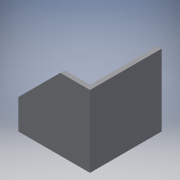
# Autodesk Inventor part: bottom left rail gusset
Saved by Autodesk Inventor 2016 (Build 200138000, 138)
## iProperties
Created: 2016-02-08
Part Number: bottom left rail gusset
Material: Aluminum 6061
Document SubType Name: Modeling
Designer: gus
Density: 2.7 g/cm^3
Appearance: Aluminum - Flat
Mass: 35.9431 g
Surface Area: 95.0795 cm^2
Volume: 13.3122 cm^3
Author: gus
Autodesk Inventor part; units mm, degrees
ref_plane "YZ Plane" through (0, 0, 0) normal (1, 0, 0) x (0, 1, 0)
ref_plane "XZ Plane" through (0, 0, 0) normal (0, 1, 0) x (-1, 0, 0)
ref_plane "XY Plane" through (0, 0, 0) normal (0, 0, 1) x (1, 0, 0)
sketch "Sketch1" plane through (0, 0, 0) normal (0, 0, 1) x (1, 0, 0)
  line L0 (0, 0) -> (0, 21.042)
  line L1 (0, 21.042) -> (29.758, 50.8)
  line L2 (29.758, 50.8) -> (50.8, 50.8)
  line L3 (50.8, 50.8) -> (50.8, 0)
  line L4 (50.8, 0) -> (0, 0)
  dimension "d0" = 50.8
  dimension "d2" = 50.8
  dimension "d3" = 50.8
  dimension "d4" = 135
  constraints: 10 end point, 3 perpendicular, 1 vertical
  measures "d0" distance of L3.end L0.start
  measures "d2" distance of L2.end L3.end
  measures "d3" distance from line of L3.end L1
  measures "d4" angle of L2 L1
extrude "Extrusion1" add sketch "Sketch1" along normal blind 3.175
sketch "Sketch2" plane through (0, 0, 3.175) normal (0, 0, 1) x (1, 0, 0)
  line L0 (50.8, 0) -> (50.8, 50.8) projected
  line L1 (0, 0) -> (50.8, 0) projected
  line L2 (50.8, 50.8) -> (47.625, 50.8)
  line L3 (47.625, 50.8) -> (47.625, 0)
  line L4 (47.625, 0) -> (50.8, 0)
  line L5 (50.8, 0) -> (50.8, 50.8)
  dimension "d7" = 3.175
  constraints: 8 end point, 2 parallel, 1 horizontal, 1 perpendicular, 1 point on line
  measures "d7" distance between parallel lines of L3 L0
extrude "Extrusion2" add sketch "Sketch2" against normal blind 50.8
sketch "Sketch3" plane through (50.8, 0, 3.175) normal (1, 0, 0) x (0, 0, -1)
  circle A0 centre (38.1, 36.9316) radius 3.3734
  circle A1 centre (12.7, 36.9316) radius 3.3734
  line L0 (0, 50.8) -> (50.8, 50.8) projected
  line L1 (0, 0) -> (0, 50.8) projected
  point P0 (3.175, 0)
  dimension "d10" = 6.7469
  dimension "d11" = 6.7469
  dimension "d12" = 13.8684
  dimension "d13" = 13.8684
  dimension "d14" = 12.7
  dimension "d15" = 25.4
  constraints: 2 centre point
  measures "d10" diameter of A0
  measures "d11" diameter of A1
  measures "d12" distance from line of A1.centre L0
  measures "d13" distance from line of L0 A0.centre
  measures "d14" distance from line of L1 A1.centre
  measures "d15" distance of A0.centre A1.centre
extrude "Extrusion3" cut sketch "Sketch3" against normal blind 3.175
sketch "Sketch4" plane through (0, 0, 0) normal (0, 0, -1) x (-1, 0, 0)
  line L0 (0, 0) -> (0, 21.042) projected
  line L1 (0, 21.042) -> (-21.042, 0)
  line L2 (-47.625, 0) -> (0, 0) projected
  line L3 (0, 21.042) -> (-29.758, 50.8) projected
  line L4 (0, 21.042) -> (0, 0)
  line L5 (-21.042, 0) -> (0, 0)
  circle A0 centre (-20.7624, 23.8439) radius 3.3734
  circle A1 centre (-38.7229, 41.8044) radius 3.3734
  dimension "d18" = 16.6624
  dimension "d19" = 12.7
  dimension "d20" = 12.7
  dimension "d21" = 6.7469
  dimension "d22" = 25.4
  constraints: 6 end point, 2 centre point, 1 equal radius, 1 horizontal, 1 perpendicular, 1 point on line, 1 vertical
  measures "d18" distance from line of A0.centre L1
  measures "d19" distance from line of L3 A0.centre
  measures "d20" distance from line of L3 A1.centre
  measures "d21" diameter of A1
  measures "d22" distance of A1.centre A0.centre
extrude "Extrusion4" cut sketch "Sketch4" against normal blind 3.175
body "Solid1"
